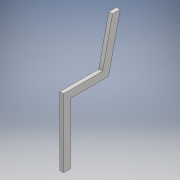
# Autodesk Inventor part: Pièce2
Saved by Autodesk Inventor 2017 (Build 210142000, 142)
## iProperties
Part Number: Pièce2
Material: Générique
Document SubType Name: Modeling
Designer: Thomas
Density: 1 g/cm^3
Appearance: Par défaut
Author: Thomas
Autodesk Inventor part; units mm, degrees
ref_plane "YZ Plane" through (0, 0, 0) normal (1, 0, 0) x (0, 1, 0)
ref_plane "XZ Plane" through (0, 0, 0) normal (0, 1, 0) x (-1, 0, 0)
ref_plane "XY Plane" through (0, 0, 0) normal (0, 0, 1) x (1, 0, 0)
sketch "Esquisse1" plane through (0, 0, 0) normal (1, 0, 0) x (0, 1, 0)
  circle A0 centre (0, 0) radius 22.5 construction
  line L0 (24.5829, 26.4096) -> (-25.4171, 26.4096)
  line L1 (-25.4171, 26.4096) -> (-25.4171, -53.5904)
  line L2 (24.5829, 26.4096) -> (39.9583, 94.7002)
  line L3 (39.9583, 94.7002) -> (29.9583, 94.7002)
  line L4 (29.9583, 94.7002) -> (16.7794, 36.1654)
  line L5 (16.7794, 36.1654) -> (-34.3848, 36.1654)
  line L6 (-34.3848, 36.1654) -> (-34.3848, -53.5904)
  line L7 (-34.3848, -53.5904) -> (-25.4171, -53.5904)
  dimension "d0" = 45
  dimension "d1" = 50
  dimension "d2" = 80
  dimension "d3" = 70
  dimension "d4" = 10
  dimension "d5" = 60
  dimension "d6" = 102.688
  dimension "d7" = 102.688
  dimension "d8" = 51.1642
  constraints: 16 end point, 2 horizontal, 2 parallel, 2 perpendicular, 1 centre point, 1 coincident
  measures "d0" diameter of A0
  measures "d1" distance of L0.start L0.end
  measures "d2" distance of L0.end L1.end
  measures "d3" distance of L0.start L2.end
  measures "d4" distance of L2.end L3.end
  measures "d5" distance of L3.end L4.end
  measures "d6" angle of L0 L2
  measures "d7" angle of L5 L4
  measures "d8" distance of L4.end L5.end
extrude "Extrusion1" add sketch "Esquisse1" along normal blind 5
